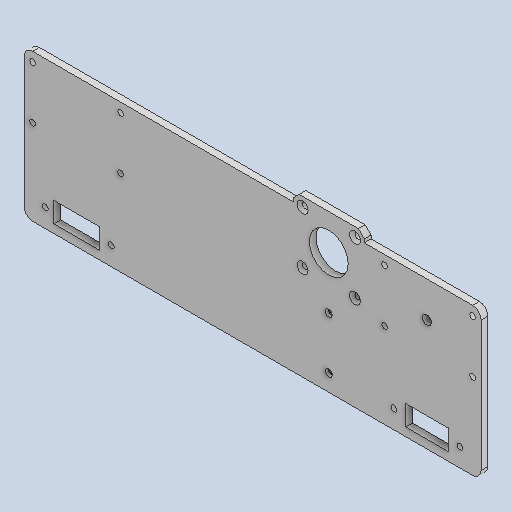
# Autodesk Inventor part: plate_2
Saved by Autodesk Inventor 2024 (Build 280153000, 153)
## iProperties
Created: 2026-02-04
Part Number: plate_2
Material: Generic
Document SubType Name: Modeling
Designer: SEMEN
Density: 1 g/cm^3
Appearance: Default
Author: SEMEN
Autodesk Inventor part; units mm, degrees
ref_plane "YZ Plane" through (0, 0, 0) normal (1, 0, 0) x (0, 1, 0)
ref_plane "XZ Plane" through (0, 0, 0) normal (0, 1, 0) x (-1, 0, 0)
ref_plane "XY Plane" through (0, 0, 0) normal (0, 0, 1) x (1, 0, 0)
sketch "Sketch1" plane through (0, 0, 0) normal (0, 0, 1) x (1, 0, 0)
  arc A0 (235.6827, -57.867) -> (240.6827, -52.867) centre (235.6827, -52.867) ccw projected
  line L0 (240.6827, -52.867) -> (240.6827, 24.133) projected
  arc A1 (240.6827, 24.133) -> (235.6827, 29.133) centre (235.6827, 24.133) ccw projected
  line L1 (235.6827, 29.133) -> (-24.3173, 29.133) projected
  arc A2 (-24.3173, 29.133) -> (-29.3173, 24.133) centre (-24.3173, 24.133) ccw projected
  line L2 (-29.3173, 24.133) -> (-29.3173, -52.867) projected
  arc A3 (-29.3173, -52.867) -> (-24.3173, -57.867) centre (-24.3173, -52.867) ccw projected
  line L3 (-24.3173, -57.867) -> (235.6827, -57.867) projected
  circle A4 centre (235.6827, 23.633) radius 1.7 projected
  circle A5 centre (235.6827, -7.367) radius 1.7 projected
  circle A6 centre (-24.3173, -7.367) radius 1.7 projected
  circle A7 centre (-24.3173, 23.633) radius 1.7 projected
  circle A8 centre (208.6827, 8.133) radius 2.75 projected
  circle A9 centre (228.1827, -46.867) radius 3.3 projected
  circle A10 centre (189.1827, -46.867) radius 3.3 projected
  circle A11 centre (22.1827, -46.867) radius 3.3 projected
  circle A12 centre (-16.8173, -46.867) radius 3.3 projected
  circle A13 centre (235.6827, -7.367) radius 1.7 projected
  circle A14 centre (235.6827, 23.633) radius 1.7 projected
  circle A15 centre (-24.3173, 23.633) radius 1.7 projected
  circle A16 centre (-24.3173, -7.367) radius 1.7 projected
  arc A17 (235.6827, -57.867) -> (240.6827, -52.867) centre (235.6827, -52.867) ccw projected
  line L4 (240.6827, -52.867) -> (240.6827, 24.133) projected
  arc A18 (240.6827, 24.133) -> (235.6827, 29.133) centre (235.6827, 24.133) ccw projected
  line L5 (235.6827, 29.133) -> (172.1827, 29.133) projected
  arc A19 (-24.3173, 29.133) -> (-29.3173, 24.133) centre (-24.3173, 24.133) ccw projected
  line L6 (-29.3173, 24.133) -> (-29.3173, -52.867) projected
  arc A20 (-29.3173, -52.867) -> (-24.3173, -57.867) centre (-24.3173, -52.867) ccw projected
  line L7 (-24.3173, -57.867) -> (235.6827, -57.867) projected
  circle A21 centre (17.1827, -7.367) radius 3.3 projected
  circle A22 centre (17.1827, 23.633) radius 3.3 projected
  circle A23 centre (-13.8173, 23.633) radius 3.3 projected
  circle A24 centre (-13.8173, -7.367) radius 3.3 projected
  circle A25 centre (208.6827, 8.133) radius 2.75 projected
  circle A26 centre (1.6827, 8.133) radius 11.5 projected
  line L8 (221.1827, -40.867) -> (221.1827, -52.867) projected
  line L9 (221.1827, -52.867) -> (196.1827, -52.867) projected
  line L10 (196.1827, -52.867) -> (196.1827, -40.867) projected
  line L11 (196.1827, -40.867) -> (221.1827, -40.867) projected
  line L12 (-11.8173, -52.867) -> (-11.8173, -40.867) projected
  line L13 (-11.8173, -40.867) -> (15.1827, -40.867) projected
  line L14 (15.1827, -40.867) -> (15.1827, -52.867) projected
  line L15 (15.1827, -52.867) -> (-11.8173, -52.867) projected
  circle A27 centre (183.6827, 23.633) radius 1.7 projected
  circle A28 centre (183.6827, -7.367) radius 1.7 projected
  circle A29 centre (27.6827, -7.367) radius 1.7 projected
  circle A30 centre (27.6827, 23.633) radius 1.7 projected
  line L16 (172.1827, 29.133) -> (172.1827, -4.0741) projected
  line L17 (172.1827, -4.0741) -> (168.3898, -7.867) projected
  line L18 (168.3898, -7.867) -> (132.9756, -7.867) projected
  line L19 (132.9756, -7.867) -> (129.1827, -4.0741) projected
  line L20 (129.1827, -4.0741) -> (129.1827, 29.133) projected
  line L21 (129.1827, 29.133) -> (-24.3173, 29.133) projected
extrude "Extrusion1" add sketch "Sketch1" along normal blind 4 contours L3 A3 L2 A2 L1 L20 L19 L18 L17 L16 A1 L0 A0 | L16 L17 L18 L19 L20 L1 | A4 | A5 | A6 | A7 | A8 | A9 | A10 | A11 | A12 | A21 | A22 | A23 | A24 | A26 | A27 | A28 | A29 | A30
hole "Hole1" at (-24.3173, -7.367, 0) at (-24.3173, 23.633, 0) at (235.6827, 23.633, 0) at (235.6827, -7.367, 0) at (27.6827, 23.633, 0) at (27.6827, -7.367, 0) at (183.6827, -7.367, 0) at (183.6827, 23.633, 0) direction (0, 0, 1) diameter 3.4 end through all clearance for "Countersunk Head GOST 12876-67" size "M3" standard "GOST"
hole "Hole2" at (208.6827, 8.133, 0) direction (0, 0, 1) diameter 5.5 end through all clearance for "Countersunk Head GOST 12876-67" size "M5" standard "GOST"
hole "Hole3" at (-16.8173, -46.867, 0) at (22.1827, -46.867, 0) at (189.1827, -46.867, 0) at (228.1827, -46.867, 0) direction (0, 0, 1) diameter 3.4 end through all countersink diameter 6.6 countersink angle 90 clearance for "Countersunk Head GOST 12876-67" size "M3" standard "GOST"
sketch "Sketch2" plane through (0, 0, 4) normal (0, 0, 1) x (1, 0, 0)
  circle A0 centre (166.1827, -1.867) radius 1.7 projected
  circle A1 centre (166.1827, 29.133) radius 1.7 projected
  circle A2 centre (135.1827, 29.133) radius 1.7 projected
  circle A3 centre (135.1827, -1.867) radius 1.7 projected
  circle A4 centre (150.6827, 13.633) radius 11 projected
  line L0 (168.1827, 34.633) -> (171.6827, 31.133) projected
  line L1 (168.1827, 34.633) -> (133.1827, 34.633) projected
  line L2 (129.6827, 31.133) -> (133.1827, 34.633) projected
  line L3 (129.6827, 31.133) -> (129.6827, -3.867) projected
  line L4 (133.1827, -7.367) -> (129.6827, -3.867) projected
  line L5 (133.1827, -7.367) -> (168.1827, -7.367) projected
  line L6 (171.6827, -3.867) -> (168.1827, -7.367) projected
  line L7 (171.6827, -3.867) -> (171.6827, 31.133) projected
  circle A5 centre (150.6827, 13.633) radius 11.5
  line L8 (150.6827, -7.367) -> (150.6827, -57.867)
  line L9 (-24.3173, -57.867) -> (235.6827, -57.867) projected
  line L10 (150.6827, -32.617) -> (163.331, -32.617) construction
  point P0 (0, 0)
  point P1 (150.6827, -17.367)
  point P2 (150.6827, -47.867)
  dimension "d23" = 0.5
  dimension "d35" = 10
  constraints: 4 end point, 3 point on line, 2 midpoint, 1 centre point, 1 horizontal, 1 symmetric about line, 1 vertical
  measures "d23" radial gap between concentric circles of A4 A5
  measures "d35" distance from line of L9 point (150.683, -47.867)
extrude "Extrusion2" cut sketch "Sketch2" against normal through all contours A4 | A5
sketch "Sketch3" plane through (0, 0, 4) normal (0, 0, 1) x (1, 0, 0)
  circle A0 centre (166.1827, -1.867) radius 1.7 projected
  circle A1 centre (166.1827, 29.133) radius 1.7 projected
  circle A2 centre (135.1827, 29.133) radius 1.7 projected
  circle A3 centre (135.1827, -1.867) radius 1.7 projected
  circle A4 centre (150.6827, 13.633) radius 11 projected
  line L0 (168.1827, 34.633) -> (171.6827, 31.133) projected
  line L1 (168.1827, 34.633) -> (133.1827, 34.633) projected
  line L2 (129.6827, 31.133) -> (133.1827, 34.633) projected
  line L3 (129.6827, 31.133) -> (129.6827, -3.867) projected
  line L4 (133.1827, -7.367) -> (129.6827, -3.867) projected
  line L5 (133.1827, -7.367) -> (168.1827, -7.367) projected
  line L6 (171.6827, -3.867) -> (168.1827, -7.367) projected
  line L7 (171.6827, -3.867) -> (171.6827, 31.133) projected
  line L8 (235.6827, 29.133) -> (-24.3173, 29.133) projected
  point P0 (0, 0)
  point P1 (129.6827, 29.133)
  point P2 (171.6827, 29.133)
extrude "Extrusion3" add sketch "Sketch3" against normal blind 4 contours L8 A1 | A1 L8 A2 L3 L2 L1 L0 L7 | L8 A2 picked at (166.251, 30.4471) picked at (135.251, 30.4471)
hole "Hole4" at (135.1827, -1.867, 4) at (135.1827, 29.133, 4) at (166.1827, 29.133, 4) at (166.1827, -1.867, 4) direction (0, 0, -1) diameter 3.4 end through all countersink diameter 6.6 countersink angle 90 clearance for "Countersunk Head GOST 12876-67" size "M3" standard "GOST"
sketch "Sketch4" plane through (0, 0, 0) normal (0, 0, -1) x (-1, 0, 0)
  point P0 (0, 0)
  point P1 (-150.6827, -17.367)
  point P2 (-150.6827, -47.867)
hole "Hole5" at (150.6827, -17.367, 0) at (150.6827, -47.867, 0) direction (0, 0, 1) diameter 4.3 end through all countersink diameter 8.6 countersink angle 90 clearance for "Countersunk Head GOST 12876-67" size "M4" standard "GOST"
body "Solid1"
